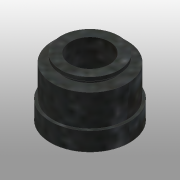
# Autodesk Inventor part: 500-107
Saved by Autodesk Inventor 2016 (Build 200138000, 138)
## iProperties
Created: 2015-04-18
Part Number: 500-107
Material: Steel
Document SubType Name: Modeling
Designer: Station9
Density: 7.85 g/cm^3
Appearance: Plate
Mass: 6.7292 g
Surface Area: 8.34954 cm^2
Volume: 0.857223 cm^3
Author: Station9
Autodesk Inventor part; units mm, degrees
ref_plane "YZ Plane" through (0, 0, 0) normal (1, 0, 0) x (0, 1, 0)
ref_plane "XZ Plane" through (0, 0, 0) normal (0, 1, 0) x (-1, 0, 0)
ref_plane "XY Plane" through (0, 0, 0) normal (0, 0, 1) x (1, 0, 0)
sketch "Sketch1" plane through (0, 0, 0) normal (0, 1, 0) x (-1, 0, 0)
  line L0 (1.7, -10.4) -> (5, -10.4)
  line L1 (5, -10.4) -> (5, -9.4)
  line L2 (3.2, -7.41) -> (1.7, -7.41)
  line L3 (1.7, -7.41) -> (1.7, -10.4)
  line L4 (5, -9.4) -> (6.408, -9.4)
  line L5 (6.408, -9.4) -> (6.408, -6.4)
  line L6 (6.408, -6.4) -> (6, -6.4)
  line L7 (3.2, 0) -> (3.2, -7.41)
  line L8 (3.2, 0) -> (6, 0)
  line L9 (6, 0) -> (6, -6.4)
  line L10 (0, 0) -> (0, -11.6607)
  dimension "d0" = 5
  dimension "d1" = 10.4
  dimension "d2" = 1
  dimension "d3" = 0
  dimension "d4" = 3
  dimension "d5" = 7.41
  dimension "d6" = 1.7
  dimension "d8" = 6
  dimension "d9" = 6.408
  dimension "d10" = 3.2
  constraints: 23 end point, 4 parallel, 2 horizontal, 2 perpendicular, 1 vertical
  measures "d0" distance between parallel lines of L10 L1
  measures "d1" distance between parallel lines of L8 L0
  measures "d2" distance between parallel lines of L0 L4
  measures "d3" distance from line of L10.start L8
  measures "d4" distance of L4.end L5.end
  measures "d5" distance between parallel lines of L8 L2
  measures "d6" distance between parallel lines of L10 L3
  measures "d8" distance between parallel lines of L10 L9
  measures "d9" distance between parallel lines of L10 L5
  measures "d10" distance between parallel lines of L10 L7
revolve "Revolution1" add sketch "Sketch1" angle 360 about axis through (0, 0, 0) along (0, 0, -1)
sketch "Sketch3" plane through (0, 0, 0) normal (1, 0, 0) x (0, 1, 0)
  line L0 (1.7, -10.4) -> (1.7, -7.41) construction
  line L1 (1.7, -7.41) -> (3.2, -7.41) construction
  line L2 (3.2, -7.41) -> (3.2, 0) construction
  line L3 (3.2, 0) -> (6, 0) construction
  line L4 (6, 0) -> (6, -6.4) construction
  line L5 (6, -6.4) -> (6.408, -6.4) construction
  line L6 (6.408, -6.4) -> (6.408, -9.4) construction
  line L7 (6.408, -9.4) -> (5, -9.4) construction
  line L8 (5, -9.4) -> (5, -10.4) construction
  line L9 (5, -10.4) -> (1.7, -10.4) construction
  line L10 (-1.7, -7.41) -> (-1.7, -10.4) construction
  line L11 (-1.7, -10.4) -> (-5, -10.4) construction
  line L12 (-5, -10.4) -> (-5, -9.4) construction
  line L13 (-5, -9.4) -> (-6.408, -9.4) construction
  line L14 (-6.408, -9.4) -> (-6.408, -6.4) construction
  line L15 (-6.408, -6.4) -> (-6, -6.4) construction
  line L16 (-6, -6.4) -> (-6, 0) construction
  line L17 (-6, 0) -> (-3.2, 0) construction
  line L18 (-3.2, 0) -> (-3.2, -7.41) construction
  line L19 (-3.2, -7.41) -> (-1.7, -7.41) construction
  line L20 (6, 0) -> (4.15, 0)
  line L21 (4.15, -0.6) -> (4.15, -1.3)
  line L22 (4.15, -1.3) -> (6, -1.3)
  line L23 (6, -1.3) -> (6, 0)
  line L24 (-6, 0) -> (6, 0) projected
  line L25 (4.15, -0.6) -> (4.75, -0.6)
  line L26 (4.75, -0.6) -> (4.75, 0)
  line L27 (4.75, 0) -> (4.15, 0)
  line L28 (0, -12.48) -> (0, 2.08) projected
  point P0 (0, 0)
  dimension "d13" = 0.6
  dimension "d14" = 1.3
  dimension "d15" = 4.15
  dimension "d16" = 4.75
  constraints: 14 end point, 3 parallel, 2 horizontal, 2 perpendicular, 1 point on line
  measures "d13" distance of L25.end L26.end
  measures "d14" distance of L20.end L21.end
  measures "d15" distance from line of point (0, 0) L21
  measures "d16" distance from line of point (0, 0) L26
revolve "Revolution2" cut sketch "Sketch3" angle 360 about axis through (0, 0, -10) along (0, 0, 1)
body "Solid1"
